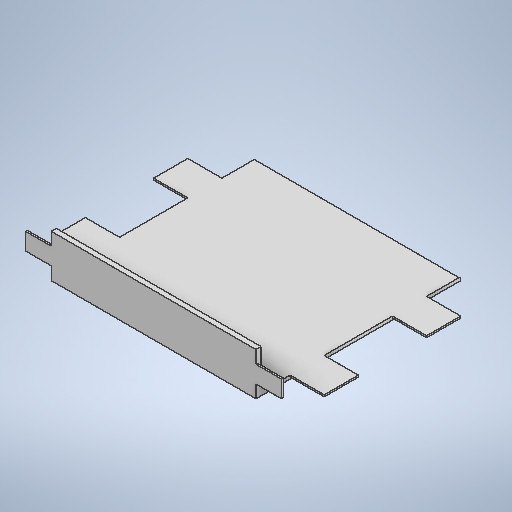
# Autodesk Inventor part: protectar1
Saved by Autodesk Inventor 2025 (Build 290162000, 162)
## iProperties
Created: 2025-11-20
Part Number: protectar1
Material: 一般
Document SubType Name: Modeling
Designer: sooo1
Density: 1 g/cm^3
Appearance: 既定
Author: sooo1
Autodesk Inventor part; units mm, degrees
ref_plane "YZ Plane" through (0, 0, 0) normal (1, 0, 0) x (0, 1, 0)
ref_plane "XZ Plane" through (0, 0, 0) normal (0, 1, 0) x (-1, 0, 0)
ref_plane "XY Plane" through (0, 0, 0) normal (0, 0, 1) x (1, 0, 0)
sketch "スケッチ1" plane through (0, 0, 0) normal (0, 1, 0) x (-1, 0, 0)
  line L0 (180, 60) -> (-180, 60)
  line L1 (-180, 60) -> (-180, -60)
  line L2 (-180, -60) -> (180, -60)
  line L3 (180, -60) -> (180, 60)
  line L4 (180, 60) -> (-180, -60) construction
  line L5 (-180, 60) -> (180, -60) construction
  line L6 (180, 57) -> (-180, 57)
  line L7 (-60, 60) -> (-60, -60)
  line L8 (-60, 40) -> (-80, 40)
  line L9 (-80, 40) -> (-80, 20)
  line L10 (-80, 20) -> (-60, 20)
  line L11 (252, 0) -> (-252, 0) construction
  line L12 (-60, -40) -> (-80, -40)
  line L13 (-80, -40) -> (-80, -20)
  line L14 (-80, -20) -> (-60, -20)
  line L15 (0, -84) -> (0, 84) construction
  line L16 (60, 60) -> (60, -60)
  line L17 (60, 40) -> (80, 40)
  line L18 (80, 40) -> (80, 20)
  line L19 (80, 20) -> (60, 20)
  line L20 (60, -40) -> (80, -40)
  line L21 (80, -20) -> (60, -20)
  line L22 (80, -40) -> (80, -20)
  line L23 (-60, 19.7) -> (-80.3, 19.7)
  line L24 (-80.3, 19.7) -> (-80.3, 40.3)
  line L25 (-80.3, 40.3) -> (-60, 40.3)
  line L26 (-60, -19.7) -> (-80.3, -19.7)
  line L27 (-80.3, -19.7) -> (-80.3, -40.3)
  line L28 (-80.3, -40.3) -> (-60, -40.3)
  line L29 (60, 19.7) -> (80.3, 19.7)
  line L30 (80.3, 19.7) -> (80.3, 40.3)
  line L31 (80.3, 40.3) -> (60, 40.3)
  line L32 (60, -19.7) -> (80.3, -19.7)
  line L33 (80.3, -19.7) -> (80.3, -40.3)
  line L34 (80.3, -40.3) -> (60, -40.3)
  point P0 (0, 0)
  point P1 (60, 57)
  point P2 (-60, 57)
  dimension "d0" = 120
  dimension "d1" = 360
  dimension "d4" = 3
  dimension "d5" = 120
  dimension "d7" = 20
  dimension "d8" = 20
  dimension "d9" = 20
  dimension "d10" = 0.3
  dimension "d11" = 0.3
  constraints: 66 end point, 22 symmetric about line, 8 point on line, 5 perpendicular, 3 horizontal, 2 midpoint, 2 parallel, 4 other
  measures "d0" distance of L0.end L1.end
  measures "d1" distance of L0.start L0.end
  measures "d4" distance between parallel lines of L0 L6
  measures "d5" distance between parallel lines of L1 L7
  measures "d7" distance of L8.end L9.end
  measures "d8" distance between parallel lines of L11 L10
  measures "d9" distance between parallel lines of L7 L9
  measures "d10" distance between parallel lines of L24 L9
  measures "d11" distance between parallel lines of L27 L13
extrude "押し出し3" add sketch "スケッチ1" along normal blind 25 contours L3 L6 L16 L0 | L16 L6 L7 L0 | L7 L6 L1 L0
sketch "スケッチ2" plane through (-180, 0, 60) normal (0, 0, 1) x (1, 0, 0)
  line L0 (0, 0) -> (360, 0) projected
  line L1 (360, 0) -> (360, 25) projected
  line L2 (0, 25) -> (360, 25) projected
  line L3 (0, 0) -> (0, 25) projected
  line L4 (240, 0) -> (240, 25)
  line L5 (240, 7.5) -> (255, 7.5)
  line L6 (255, 7.5) -> (255, 17.5)
  line L7 (255, 17.5) -> (240, 17.5)
  line L8 (180, -5) -> (180, 30) construction
  line L9 (120, 0) -> (120, 25)
  line L10 (120, 7.5) -> (105, 7.5)
  line L11 (105, 7.5) -> (105, 17.5)
  line L12 (105, 17.5) -> (120, 17.5)
  line L13 (240, 17.9) -> (255.4, 17.9)
  line L14 (255.4, 17.9) -> (255.4, 7.1)
  line L15 (255.4, 7.1) -> (240, 7.1)
  line L16 (120, 17.9) -> (104.6, 17.9)
  line L17 (104.6, 17.9) -> (104.6, 7.1)
  line L18 (104.6, 7.1) -> (120, 7.1)
  point P0 (180, 0)
  point P1 (360, 12.5)
  dimension "d16" = 120
  dimension "d17" = 10
  dimension "d18" = 15
  dimension "d19" = 7.5
  dimension "d24" = 0.4
  constraints: 28 end point, 10 symmetric about line, 6 point on line, 4 perpendicular, 1 horizontal, 1 midpoint, 2 other
  measures "d16" distance from line of point (360, 12.5) L4
  measures "d17" distance of L5.end L6.end
  measures "d18" distance of L6.end L7.end
  measures "d19" distance between parallel lines of L2 L7
  measures "d24" distance between parallel lines of L6 L14
extrude "押し出し6" add sketch "スケッチ1" along normal blind 2 contours L16 L2 L7 L6
extrude "押し出し7" add sketch "スケッチ1" against normal blind 1 from surface at 2 contours L17 L18 L19 L16 | L7 L10 L9 L8 | L16 L21 L22 L20 | L12 L13 L14 L7
extrude "押し出し8" cut sketch "スケッチ2" against normal up to surface (3 mm away) contours L3 L2 L9 L16 L17 L18 L0 | L4 L15 L14 L13 L2 L1 L0 | L18 L17 L16 L9 L12 L11 L10 | L4 L5 L6 L7 L13 L14 L15 | L10 L11 L12 L9 | L4 L7 L6 L5
fillet "フィレット2" radius 1 1 edges at (0, 2, -60)
extrude "押し出し9" add sketch "スケッチ2" against normal blind 1 contours L10 L11 L12 L9 | L4 L7 L6 L5
fillet "フィレット3" radius 4 1 edges at (0, 2, 57)
